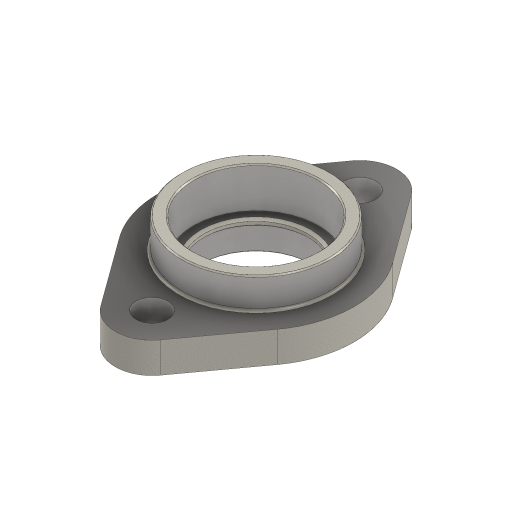
# Autodesk Inventor part: Part037. Main arbor flange
Saved by Autodesk Inventor 2023.2 (Build 272271030, 271C)
## iProperties
Created: 2023-11-17
Part Number: Part037. Main arbor flange
Material: Steel, Carbon
Document SubType Name: Modeling
Designer: User
Mass: 4223.16 g
Surface Area: 860.792 cm^2
Volume: 537.982 cm^3
Density: 7.85 g/cm^3
Appearance: Steel - Cast
Author: User
Autodesk Inventor part; units mm, degrees
note: some values were not read from the file. Chosen so that the rebuilt part matches the saved one: direction of "Hole2".
ref_plane "XZ Plane" through (0, 0, 0) normal (0, 1, 0) x (-1, 0, 0)
ref_plane "XY Plane" through (0, 0, 0) normal (0, 0, 1) x (1, 0, 0)
sketch "Sketch1" plane through (0, 0, 0) normal (0, 1, 0) x (-1, 0, 0)
  line L0 (64.6952, -47.0588) -> (24.2607, -102.6471)
  arc A0 (-24.2607, -102.6471) -> (24.2607, -102.6471) centre (0, -85) ccw
  line L1 (-24.2607, -102.6471) -> (-64.6952, -47.0588)
  arc A1 (-64.6952, 47.0588) -> (-64.6952, -47.0588) centre (0, 0) ccw
  line L2 (-64.6952, 47.0588) -> (-24.2607, 102.6471)
  arc A2 (24.2607, 102.6471) -> (-24.2607, 102.6471) centre (0, 85) ccw
  line L3 (24.2607, 102.6471) -> (64.6952, 47.0588)
  arc A3 (64.6952, -47.0588) -> (64.6952, 47.0588) centre (0, 0) ccw
  dimension "d0" = 170
  dimension "d1" = 160
  dimension "d3" = 30
  constraints: 8 end point, 8 point on circle, 8 tangent, 4 centre point, 2 coincident, 2 equal radius, 2 vertical alignment, 1 parallel
  measures "d0" distance of A2.centre A0.centre
  measures "d1" diameter of A3
  measures "d3" radius of A0
extrude "Extrusion1" add sketch "Sketch1" along normal mid plane 25
sketch "Sketch2" plane through (0, 12.5, 0) normal (0, 1, 0) x (1, 0, 0)
  arc A0 (24.2607, 102.6471) -> (-24.2607, 102.6471) centre (0, 85) ccw projected
  arc A1 (-24.2607, -102.6471) -> (24.2607, -102.6471) centre (0, -85) ccw projected
hole "Hole1" at (0, 12.5, -85) at (0, 12.5, 85) direction (0, -1, 0) diameter 26 end through all
sketch "Sketch3" plane through (0, 0, 0) normal (0, 0, 1) x (1, 0, 0)
  line L0 (0, 37.5) -> (0, -20.5)
  line L1 (0, 37.5) -> (-61, 37.5)
  line L2 (-61, 37.5) -> (-61, -12.5)
  line L3 (-64.6952, -12.5) -> (-24.2607, -12.5) projected
  line L4 (-61, -12.5) -> (-57.5, -12.5)
  line L5 (-57.5, -12.5) -> (-57.5, -20.5)
  line L6 (-57.5, -20.5) -> (0, -20.5)
  line L7 (-24.2607, 12.5) -> (-64.6952, 12.5) projected
  point P0 (0, 0)
  dimension "d13" = 58
  dimension "d14" = 122
  dimension "d15" = 115
  dimension "d16" = 25
  constraints: 12 end point, 2 horizontal, 2 perpendicular, 2 point on line, 2 vertical
  measures "d13" distance of L0.start L0.end
  measures "d14" diameter of L2 L0
  measures "d15" diameter of L5 L0
  measures "d16" distance between parallel lines of L7 L1
revolve "Revolution1" add sketch "Sketch3" angle 360 about axis through (0, 37.5, 0) along (0, -1, 0)
sketch "Sketch4" plane through (0, 0, 0) normal (0, 0, 1) x (1, 0, 0)
  line L0 (0, -20.5) -> (0, 37.5)
  line L1 (-61, 37.5) -> (61, 37.5) projected
  line L2 (0, 37.5) -> (-51, 37.5)
  line L3 (-51, 37.5) -> (-51, 4.5)
  line L4 (-51, 4.5) -> (-45, 4.5)
  line L5 (-42.5, 3) -> (-42.5, -0.5)
  line L6 (-42.5, -0.5) -> (-45, -0.5)
  line L7 (-45, -0.5) -> (-45, -20.5)
  line L8 (-57.5, -20.5) -> (57.5, -20.5) projected
  line L9 (-45, -20.5) -> (0, -20.5)
  line L10 (-45, 4.5) -> (-42.5, 3)
  point P0 (0, 0)
  dimension "d18" = 102
  dimension "d19" = 90
  dimension "d20" = 85
  dimension "d21" = 33
  dimension "d22" = 20
  dimension "d23" = 1.5
  dimension "d24" = 90
  constraints: 18 end point, 5 perpendicular, 3 point on line, 1 midpoint, 1 vertical
  measures "d18" diameter of L3 L0
  measures "d19" diameter of L7 L0
  measures "d20" diameter of L5 L0
  measures "d21" distance between parallel lines of L1 L4
  measures "d22" distance between parallel lines of L8 L6
  measures "d23" distance from line of L4 L5.start
  measures "d24" diameter of L4.end L0
revolve "Revolution2" cut sketch "Sketch4" angle 360 about axis through (0, -20.5, 0) along (0, 1, 0)
hole "Hole2" at (-69.282, -0.5, 40) direction (0.8660254, 0, -0.5) diameter 6 end up to surface
hole "Hole3" at (-69.282, -0.5, 40) direction (0.8660254, 0, -0.5) diameter 11.445 depth 18 tip angle 118
thread "Thread1" size "G13.157x1.337" designation "G 1/4" standard "ISO Pipe Threads" length 14
sketch "Sketch5" plane through (0, -12.5, 0) normal (0, -1, 0) x (1, 0, 0)
  arc A0 (64.6952, -47.0588) -> (64.6952, 47.0588) centre (0, 0) ccw projected
  line L0 (0, 0) -> (47.7297, 47.7297) construction
  line L1 (0, 0) -> (67.5, 0) construction
  dimension "d48" = 67.5
  dimension "d49" = 45
  constraints: 4 end point, 1 coincident, 1 equal length, 1 horizontal
  measures "d48" distance of L0.start L0.end
  measures "d49" angle of L1 L0
hole "Hole4" at (47.7297, -12.5, 47.7297) direction (0, 1, 0) diameter 8.376 depth 18 tip angle 118 thread size "M10x1.5" class "6H" standard "ISO Metric profile"
pattern_circular "Circular Pattern1" count 4 over 360 about axis through (0, -16.5, 0) along (0, -1, 0) of "Hole4"
fillet "Fillet1" radius 2 2 edges at (61, 12.5, 0) (57.5, -12.5, 0)
chamfer "Chamfer1" distance 1 angle 45 6 edges at (57.5, -20.5, 0) (45, -20.5, 0) (61, 37.5, 0) (51, 37.5, 0) (-41.4147, -0.5, 9.5432) (40.6378, -0.5, -12.4427)
ref_plane "Work Plane1" through (0, -0.5, 0) normal (0, 1, 0) x (1, 0, 0)
ref_plane "Work Plane2" through (0, 0, 0) normal (-0.5, 0, -0.8660254) x (0, 1, 0)
body "Solid1"
